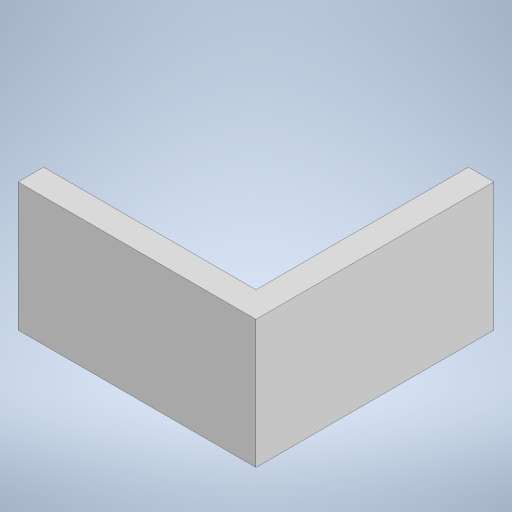
# Autodesk Inventor part: TestingPlatform_stackFeet01
Saved by Autodesk Inventor 2024.2 (Build 282272000, 272)
## iProperties
Created: 2024-01-30
Part Number: TestingPlatform_stackFeet01
Material: Generic
Document SubType Name: Modeling
Designer: ringl
Density: 1 g/cm^3
Appearance: Default
Author: ringl
Autodesk Inventor part; units mm, degrees
ref_plane "YZ Plane" through (0, 0, 0) normal (1, 0, 0) x (0, 1, 0)
ref_plane "XZ Plane" through (0, 0, 0) normal (0, 1, 0) x (-1, 0, 0)
ref_plane "XY Plane" through (0, 0, 0) normal (0, 0, 1) x (1, 0, 0)
sketch "Sketch1" plane through (0, 0, 0) normal (0, 1, 0) x (-1, 0, 0)
  line L0 (0, 0) -> (16.7, 0)
  line L1 (16.7, 0) -> (16.7, -4)
  line L2 (16.7, -4) -> (4, -4)
  line L3 (4, -4) -> (4, -16.7)
  line L4 (4, -16.7) -> (0, -16.7)
  line L5 (0, -16.7) -> (0, 0)
  dimension "d0" = 16.7
  dimension "d1" = 4
  dimension "d2" = 4
  dimension "d3" = 16.7
  constraints: 12 end point, 5 perpendicular, 1 horizontal
  measures "d0" distance of L0.start L0.end
  measures "d1" distance of L0.end L1.end
  measures "d2" distance of L3.end L4.end
  measures "d3" distance of L4.end L0.start
extrude "Extrusion1" add sketch "Sketch1" along normal blind 5
sketch "Sketch2" plane through (0, 5, 0) normal (0, 1, 0) x (1, 0, 0)
  line L0 (-16.7, 4) -> (-16.7, 0) projected
  line L1 (-16.7, 0) -> (-16.7, 1.8)
  line L2 (-16.7, 1.8) -> (-1.8, 1.8)
  line L3 (-1.8, 1.8) -> (-1.8, 16.7)
  line L4 (-1.8, 16.7) -> (0, 16.7)
  line L5 (-16.7, 0) -> (0, 0) projected
  line L6 (0, 16.7) -> (0, 0)
  line L7 (-16.7, 0) -> (0, 0)
  dimension "d6" = 1.8
  dimension "d7" = 1.8
  dimension "d8" = 16.7
  constraints: 12 end point, 4 perpendicular, 1 collinear, 1 point on line
  measures "d6" distance of L0.end L1.end
  measures "d7" distance of L3.end L4.end
  measures "d8" distance of L4.end L5.end
extrude "Extrusion2" add sketch "Sketch2" along normal blind 4
body "Solid1"
